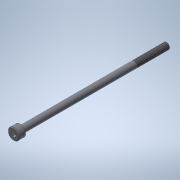
# Autodesk Inventor part: SCREW, SOCKET HD, P, 12.9, M4X0.7X90MM
Saved by Autodesk Inventor 2022.4 (Build 264492000, 492)
## iProperties
Category: _
Manager: 100-20545
Created: 2023-03-10
Part Number: SCREW, SOCKET HD, P, 12.9, M4X0.7X90MM
Checked By: 0003881535
Engr Approved By: P
User Status: Released
Material: Steel, MS
Description: SCREW, SOCKET HD, P, 12.9, M4X0.7X90MM
Document SubType Name: Modeling
Mfg Approved By: Cathy.Lesperance
Designer: Clint.Matte
Manufacturer: Standard
Standards Organization: Custom
Density: 7.86 g/cm^3
Appearance: Metal-Steel
Mass: 9.96167 g
Surface Area: 13.0981 cm^2
Volume: 1.26739 cm^3
CN_MASS: 0.01
CN_SERVICEABLE: _
FIRST_DESCRIPTION: SCREW, SOCKET HD, P, 12.9, M4X0.7X90MM
SECOND_DESCRIPTION: _
THIRD_DESCRIPTION: _
ModelCat: Uncategorized
PTC_WM_ITERATION: 2
PTC_WM_ORGANIZATION_ID: CLWC
PTC_WM_LIFECYCLE: CLWC_CAD_LC
Subject: _
Author: -
Keywords: DEFAULT
Revision Number: A
Autodesk Inventor part; units mm, degrees
ref_plane "YZ Plane" through (0, 0, 0) normal (1, 0, 0) x (0, 1, 0)
ref_plane "XZ Plane" through (0, 0, 0) normal (0, 1, 0) x (-1, 0, 0)
ref_plane "XY Plane" through (0, 0, 0) normal (0, 0, 1) x (1, 0, 0)
sketch "Sketch3" plane through (0, 0, 0) normal (0, 0, 1) x (1, 0, 0)
  circle A0 centre (0, 0) radius 2
  dimension "Diameter" = 4
  constraints: 1 centre point, 1 coincident
  measures "Diameter" diameter of A0
extrude "Extrusion1" add sketch "Sketch3" against normal blind 90
sketch "Sketch4" plane through (0, 0, 0) normal (0, 0, 1) x (1, 0, 0)
  circle A0 centre (0, 0) radius 2 projected
  circle A1 centre (0, 0) radius 3.5
  dimension "Head_Diameter" = 7
  constraints: 1 centre point, 1 coincident
  measures "Head_Diameter" diameter of A1
extrude "Extrusion2" add sketch "Sketch4" along normal blind 4 contours A0 | A1
sketch "Sketch5" plane through (0, 0, 4) normal (0, 0, 1) x (1, 0, 0)
  circle A0 centre (0, 0) radius 3.5 projected
  line L0 (1.7321, 0) -> (0.866, -1.5)
  line L1 (0.866, -1.5) -> (-0.866, -1.5)
  line L2 (-0.866, -1.5) -> (-1.7321, 0)
  line L3 (-1.7321, 0) -> (-0.866, 1.5)
  line L4 (-0.866, 1.5) -> (0.866, 1.5)
  line L5 (0.866, 1.5) -> (1.7321, 0)
  line L6 (0, 0) -> (1.7321, 0) construction
  dimension "Hex_Width" = 3
  constraints: 14 end point, 1 coincident, 1 horizontal, 13 other
  measures "Hex_Width" distance between parallel lines of L1 L4
extrude "Extrusion3" cut sketch "Sketch5" against normal blind 2 contours L0 L1 L2 L3 L4 L5
thread "Thread1" size "M4x0.7" class "4g6g" standard "ANSI Metric M Profile" length 20
chamfer "Chamfer1" distance 0.4 angle 45 1 edges at (-3.5, 0, 4)
chamfer "Chamfer2" distance 0.2 angle 45 1 edges at (-2, 0, -90)
equation "\"d14\" = 0.5 * Chamfer"
equation "\"Chamfer\" = 0.4"
body "Solid1"
